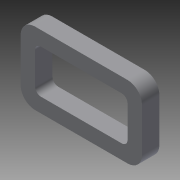
# Autodesk Inventor part: Center Block
Saved by Autodesk Inventor 2013 SP1 (Build 170176100, 176)
## iProperties
Created: 2013-08-06
Part Number: Center Block
Material: Generic
Document SubType Name: Modeling
Designer: Eric
Density: 1 g/cm^3
Author: Eric
Autodesk Inventor part; units mm, degrees
ref_plane "YZ Plane" through (0, 0, 0) normal (1, 0, 0) x (0, 1, 0)
ref_plane "XZ Plane" through (0, 0, 0) normal (0, 1, 0) x (-1, 0, 0)
ref_plane "XY Plane" through (0, 0, 0) normal (0, 0, 1) x (1, 0, 0)
sketch "Sketch1" plane through (0, 0, 0) normal (0, 1, 0) x (-1, 0, 0)
  line L0 (2, 0) -> (30, 0)
  line L1 (32, 2) -> (32, 13)
  line L2 (30, 15) -> (2, 15)
  line L3 (0, 13) -> (0, 2)
  line L4 (0, 20) -> (32, 20)
  line L5 (37, 15) -> (37, 0)
  line L6 (32, -5) -> (0, -5)
  line L7 (-5, 0) -> (-5, 15)
  arc A0 (0, 20) -> (-5, 15) centre (0, 15) ccw
  arc A1 (37, 15) -> (32, 20) centre (32, 15) ccw
  arc A2 (32, -5) -> (37, 0) centre (32, 0) ccw
  arc A3 (-5, 0) -> (0, -5) centre (0, 0) ccw
  arc A4 (2, 15) -> (0, 13) centre (2, 13) ccw
  arc A5 (32, 13) -> (30, 15) centre (30, 13) ccw
  arc A6 (30, 0) -> (32, 2) centre (30, 2) ccw
  arc A7 (0, 2) -> (2, 0) centre (2, 2) ccw
  point P0 (0, 0)
  point P1 (32, 0)
  point P2 (0, 15)
  dimension "d0" = 15
  dimension "d1" = 32
  dimension "d2" = 5
  dimension "d3" = 5
  dimension "d4" = 5
  dimension "d5" = 5
  dimension "d6" = 5
  dimension "d7" = 2
  constraints: 16 end point, 16 point on circle, 16 tangent, 8 centre point, 6 equal radius, 6 point on line, 4 parallel, 2 horizontal, 2 perpendicular
  measures "d0" distance of point (0, 15) point (0, 0)
  measures "d1" distance of point (0, 0) point (32, 0)
  measures "d2" distance between parallel lines of L5 L1
  measures "d3" distance between parallel lines of L4 L2
  measures "d4" distance between parallel lines of L7 L3
  measures "d5" distance between parallel lines of L6 L0
  measures "d6" radius of A0
  measures "d7" radius of A4
extrude "Extrusion1" add sketch "Sketch1" along normal blind 6
body "Solid1"
